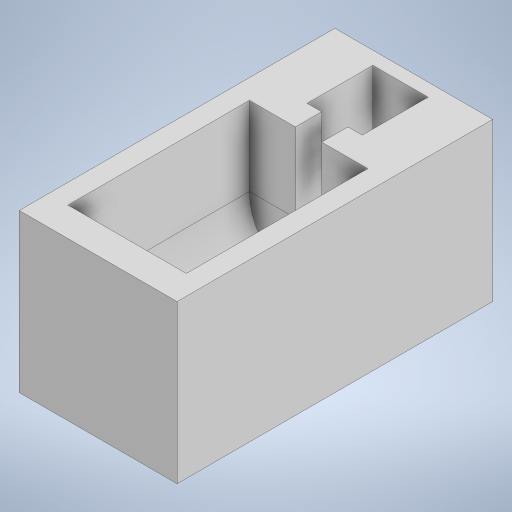
# Autodesk Inventor part: housing_V2
Saved by Autodesk Inventor 2023 (Build 270158000, 158)
## iProperties
Created: 2023-03-23
Part Number: housing_V2
Material: Generic
Document SubType Name: Modeling
Designer: caleb
Density: 1 g/cm^3
Appearance: Default
Author: caleb
Autodesk Inventor part; units mm, degrees
ref_plane "YZ Plane" through (0, 0, 0) normal (1, 0, 0) x (0, 1, 0)
ref_plane "XZ Plane" through (0, 0, 0) normal (0, 1, 0) x (-1, 0, 0)
ref_plane "XY Plane" through (0, 0, 0) normal (0, 0, 1) x (1, 0, 0)
sketch "Sketch1" plane through (0, 0, 0) normal (0, 1, 0) x (-1, 0, 0)
  line L0 (-0.0661, 0.1517) -> (59.9339, 0.1517)
  line L1 (59.9339, 0.1517) -> (59.9339, -119.8483)
  line L2 (59.9339, -119.8483) -> (-0.0661, -119.8483)
  line L3 (-0.0661, -119.8483) -> (-0.0661, 0.1517)
  line L4 (29.9339, -119.8483) -> (29.9339, 0.1517)
  circle A0 centre (29.9339, -54.8547) radius 22.5
  line L5 (19.5008, -89.8484) -> (19.5008, -114.8484)
  line L6 (19.5008, -114.8484) -> (40.5008, -114.8484)
  line L7 (40.5008, -114.8484) -> (40.5008, -89.8484)
  line L8 (40.5008, -89.8484) -> (19.5008, -89.8484)
  line L9 (19.5008, -89.8484) -> (40.5008, -114.8484) construction
  line L10 (19.5008, -114.8484) -> (40.5008, -89.8484) construction
  line L11 (19.5008, -89.8484) -> (44.5008, -89.8484) construction
  line L12 (24.9546, -79.8533) -> (24.9546, -89.8533)
  line L13 (24.9546, -89.8533) -> (34.9546, -89.8533)
  line L14 (34.9546, -89.8533) -> (34.9546, -79.8533)
  line L15 (34.9546, -79.8533) -> (24.9546, -79.8533)
  line L16 (24.9546, -79.8533) -> (34.9546, -89.8533) construction
  line L17 (24.9546, -89.8533) -> (34.9546, -79.8533) construction
  line L18 (24.9546, -79.8533) -> (34.9546, -79.8533) construction
  line L19 (7.4339, -10.8533) -> (7.4339, -79.8533)
  line L20 (7.4339, -79.8533) -> (52.4339, -79.8533)
  line L21 (52.4339, -79.8533) -> (52.4339, -10.8533)
  line L22 (52.4339, -10.8533) -> (7.4339, -10.8533)
  line L23 (7.4339, -10.8533) -> (52.4339, -79.8533) construction
  line L24 (7.4339, -79.8533) -> (52.4339, -10.8533) construction
  line L25 (7.4339, -10.8533) -> (76.4339, -10.8533) construction
  point P0 (0, 0)
  point P1 (29.9339, -114.8483)
  point P2 (30.4342, -89.8533)
  point P3 (29.9546, -89.8533)
  point P4 (29.9339, -79.8533)
  point P5 (30.0136, -77.3546)
  point P6 (29.9339, -25)
  point P7 (30.0008, -102.3484)
  point P8 (29.9339, -10.8533)
  point P9 (29.9546, -84.8533)
  point P10 (29.9339, -10.8533)
  point P11 (29.9339, -45.3533)
  point P12 (34.9546, -79.8533)
  point P13 (24.9546, -79.8533)
  point P14 (24.9546, -89.8484)
  point P15 (34.9546, -89.8484)
  dimension "d0" = 60
  dimension "d1" = 120
  dimension "d2" = 45
  dimension "d3" = 5
  dimension "d4" = 25
  dimension "d6" = 12.5
  dimension "d7" = 10
  dimension "d8" = 2.5
  dimension "d9" = 22.5
  dimension "d10" = -69
  dimension "d11" = 25
  dimension "d12" = 90
  dimension "d13" = 21
  dimension "d14" = 5
  dimension "d15" = 10
  dimension "d16" = 90
  dimension "d17" = 10
  dimension "d18" = -69
  dimension "d19" = 90
  dimension "d20" = -34.5
  dimension "d21" = 45
  constraints: 52 end point, 11 parallel, 9 midpoint, 7 perpendicular, 6 point on line, 4 horizontal, 2 coincident, 1 centre point
  measures "d0" distance of L2.start L2.end
  measures "d1" distance of L1.start L2.start
  measures "d2" diameter of A0
  measures "d3" distance from line of L2 point (29.934, -114.848)
  measures "d4" distance of point (30.434, -89.853) point (29.934, -114.848)
  measures "d6" distance of point (29.934, -114.848) point (30.001, -102.348)
  measures "d7" distance of point (29.934, -79.853) point (29.955, -89.853)
  measures "d8" distance of point (30.014, -77.355) point (29.934, -79.853)
  measures "d9" distance of point (29.934, -54.855) point (30.014, -77.355)
  measures "d10" distance of point (29.934, -10.853) point (29.934, -79.853)
  measures "d11" distance of L8.end L5.end
  measures "d12" angle of L5 L11
  measures "d13" distance of L7.start L5.end
  measures "d14" distance of point (29.955, -84.853) point (29.955, -89.853)
  measures "d15" distance of L15.end L12.end
  measures "d16" angle of L12 L18
  measures "d17" distance of L14.start L12.end
  measures "d18" distance of L19.start L20.start
  measures "d19" angle of L19 L25
  measures "d20" distance of point (29.934, -79.853) point (29.934, -45.353)
  measures "d21" distance between parallel lines of L19 L21
extrude "Extrusion1" add sketch "Sketch1" against normal blind 60
sketch "Sketch2" plane through (0.0661, 0, -119.8483) normal (0, 0, -1) x (-1, 0, 0)
  line L0 (0, 0) -> (60, 0) projected
  line L1 (0, 0) -> (0, -60) projected
  line L2 (60, -60) -> (0, -60) projected
  line L3 (60, 0) -> (60, -60) projected
  point P0 (0.0661, 0)
  point P1 (30, -30)
ref_plane "Work Plane1" through (-19.5008, 0, -114.8484) normal (0, 0, -1) x (-1, 0, 0)
ref_plane "Work Plane2" through (-19.5008, 0, -89.8484) normal (0, 0, -1) x (-1, 0, 0)
ref_plane "Work Plane3" through (-24.9546, 0, -79.8533) normal (0, 0, -1) x (-1, 0, 0)
ref_plane "Work Plane5" through (-7.4339, 0, -5.8533) normal (0, 0, -1) x (-1, 0, 0)
ref_plane "Work Plane4" through (-7.4339, 0, -10.8533) normal (0, 0, -1) x (-1, 0, 0)
sketch "Sketch3" plane through (-19.5008, 0, -114.8484) normal (0, 0, -1) x (-1, 0, 0)
  circle A0 centre (10.433, -30) radius 10.5
  point P0 (-19.5008, 0)
  dimension "d25" = 21
  constraints: 1 centre point, 1 coincident
  measures "d25" diameter of A0
ref_plane "Work Plane6" through (-29.9339, -30, -119.8483) normal (0, 1, 0) x (1, 0, 0)
extrude "Extrusion3" cut sketch "Sketch1" against normal up to surface (30 mm away) contours L22 L21 A0 L4 | L4 A0 L19 L22 | A0 L4 | L4 A0 | L6 L5 L8 L12 L13 L4 | L4 L13 L14 L8 L7 L6 | A0 L21 L20 L15 L4 | L4 L15 L20 L19 A0 | L13 L12 L8 L4 | L4 L8 L14 L13 | L15 L14 L8 L4 | L4 L8 L12 L15
sketch "Sketch4" plane through (-19.5008, 0, -89.8484) normal (0, 0, -1) x (-1, 0, 0)
  circle A0 centre (10.433, -30) radius 5
  point P0 (-19.5008, 0)
  point P1 (15.4537, 0)
  point P2 (15.4537, 0)
  point P3 (15.4537, 0)
  point P4 (5.4537, 0)
  point P5 (5.4537, 0)
  point P6 (5.4537, 0)
  dimension "d30" = 10
  constraints: 1 centre point, 1 coincident
  measures "d30" diameter of A0
sketch "Sketch5" plane through (-24.9546, 0, -79.8533) normal (0, 0, -1) x (-1, 0, 0)
  circle A0 centre (4.9793, -30) radius 22.5
  point P0 (-24.9546, 0)
  dimension "d31" = 45
  constraints: 1 centre point, 1 coincident
  measures "d31" diameter of A0
extrude "Extrusion4" cut sketch "Sketch3" against normal up to surface (25 mm away)
ref_plane "Work Plane7" through (0.0661, 0, -117.8483) normal (0, 0, -1) x (-1, 0, 0)
extrude "Extrusion5" cut sketch "Sketch4" against normal up to surface (83.9952 mm away)
extrude "Extrusion6" cut sketch "Sketch5" against normal up to surface (69 mm away)
extrude "Extrusion7" cut sketch "Sketch4" along normal up to surface (27.9998 mm away)
equation "\"d4\" = d11"
equation "\"d6\" = 0.5 * d4"
equation "\"d7\" = d15"
equation "\"d9\" = 0.5 * d2"
equation "\"d14\" = 0.5 * d7"
equation "\"d18\" = d10"
equation "\"d20\" = 0.5 * d10"
equation "\"d21\" = d2"
equation "\"d31\" = d2"
body "Solid1"
